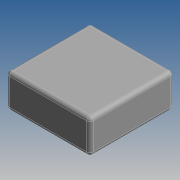
# Autodesk Inventor part: FE016
Saved by Autodesk Inventor 2015 SP1 (Build 190203100, 203)
## iProperties
Created: 2014-10-07
Part Number: FE016
Material: Fourniture / Geliefertes
Document SubType Name: Modeling
Designer: grp
Density: 1 g/cm^3
Appearance: Par défaut
Description: Aimant
Author: grp
Autodesk Inventor part; units mm, degrees
ref_plane "YZ Plane" through (0, 0, 0) normal (1, 0, 0) x (0, 1, 0)
ref_plane "XZ Plane" through (0, 0, 0) normal (0, 1, 0) x (-1, 0, 0)
ref_plane "XY Plane" through (0, 0, 0) normal (0, 0, 1) x (1, 0, 0)
sketch "Sketch1" plane through (0, 0, 0) normal (0, 0, 1) x (1, 0, 0)
  line L0 (0, 0) -> (5, 0)
  line L1 (5, 0) -> (5, 5)
  line L2 (5, 5) -> (0, 5)
  line L3 (0, 5) -> (0, 0)
  dimension "d0" = 5
  dimension "d1" = 5
  constraints: 8 end point, 2 parallel, 1 horizontal, 1 perpendicular
  measures "d0" distance of L2.end L1.end
  measures "d1" distance of L1.end L0.end
extrude "Extrusion1" add sketch "Sketch1" along normal blind 2
fillet "Congé1" radius 0.2 12 edges at (2.5, 0, 2) (5, 2.5, 2) (2.5, 5, 2) (0, 2.5, 2) (2.5, 0, 0) (5, 0, 1) (0, 0, 1) (5, 2.5, 0) (5, 5, 1) (2.5, 5, 0) (0, 5, 1) (0, 2.5, 0)
